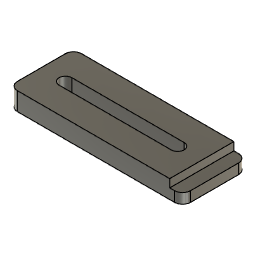
clampMekanika v3 (Autodesk Fusion 360 design; units mm, degrees)
Autodesk Fusion 360 part; units mm, degrees
sketch "Sketch3" plane through (0, 0, 0) normal (0, 0, 1) x (1, 0, 0)
  line L0 (50, -20) -> (-50, -20)
  line L1 (-50, -20) -> (-50, 20)
  line L2 (-50, 20) -> (50, 20)
  line L3 (50, 20) -> (50, -20)
  line L4 (50, -20) -> (-50, 20) construction
  line L5 (-50, -20) -> (50, 20) construction
  line L6 (35, -4) -> (-35, -4)
  line L7 (-35, -4) -> (-35, 4)
  line L8 (-35, 4) -> (35, 4)
  line L9 (35, 4) -> (35, -4)
  line L10 (35, -4) -> (-35, 4) construction
  line L11 (-35, -4) -> (35, 4) construction
  line L12 (50, 20) -> (58, 20)
  line L13 (58, 20) -> (58, -20)
  line L14 (58, -20) -> (50, -20)
  line L15 (50, -20) -> (50, 20)
  circle A0 centre (-35, 0) radius 4
  circle A1 centre (35, 0) radius 4
  dimension "d9" = 100
  dimension "d10" = 40
  dimension "d11" = 70
  dimension "d12" = 8
  dimension "d14" = 8
  dimension "d15" = 40
  dimension "d16" = 8
  dimension "d17" = 8
  constraint horizontal L0
  constraint perpendicular L0 L1
  constraint parallel L0 L2
  constraint parallel L1 L3
  constraint coincident L4 origin
  constraint coincident L5 origin
  constraint horizontal L6
  constraint perpendicular L6 L7
  constraint parallel L6 L8
  constraint parallel L7 L9
  constraint coincident L10 origin
  constraint coincident L11 origin
  constraint horizontal L12
  constraint vertical L13
  constraint horizontal L14
  constraint vertical L15
  constraint midpoint L7 A0.centre
  constraint midpoint L9 A1.centre
  measures "d9" distance of L1.end L2.end
  measures "d10" distance of L0.end L1.end
  measures "d11" distance of L7.end L8.end
  measures "d12" distance of L6.end L7.end
  measures "d14" distance of L2.end L12.end
  measures "d15" distance of L2.end L0.start
  measures "d16" diameter of A0
  measures "d17" diameter of A1
extrude "Extrude1" add sketch "Sketch3" along normal blind 11.3 contours L0 L1 L2 L3 L15
extrude "Extrude2" add sketch "Sketch3" along normal blind 6.3 contours L3 L12 L13 L14 L15
fillet "Fillet1" radius 5 4 edges at (-50, -20, 5.65) (-50, 20, 5.65) (58, 20, 3.15) (58, -20, 3.15)
equation "thickness = 11.3 mm"
equation "largeur = 40 mm"
equation "longueurTotal = 100 mm"
equation "diametre = 8 mm"
equation "epaulement = thickness - 5 mm"
equation "congés = 5 mm"
equation "longueurRainure = longueurTotal - 30 mm"
equation "largeurRainure = 8 mm"
equation "d9 = longueurTotal"
equation "d10 = largeur"
equation "d11 = longueurRainure"
equation "d12 = largeurRainure"
equation "largeurEpaulement = 8 mm"
equation "d14 = largeurEpaulement"
equation "d15 = largeur"
equation "d16 = diametre"
equation "d17 = diametre"
equation "d18 = thickness"
equation "d20 = epaulement"
equation "d23 = congés"
